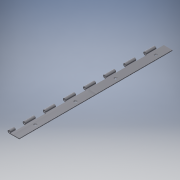
# Autodesk Inventor part: SIDE 1
Saved by Autodesk Inventor 2016 (Build 200138000, 138)
## iProperties
Created: 2015-09-17
Part Number: SIDE 1
Material: Steel, Mild
Document SubType Name: Modeling
Designer: testing
Density: 7.85 g/cm^3
Appearance: Metal-Steel
Mass: 86.1353 g
Surface Area: 160.581 cm^2
Volume: 10.9727 cm^3
Author: testing
Autodesk Inventor part; units mm, degrees
ref_plane "YZ Plane" through (0, 0, 0) normal (1, 0, 0) x (0, 1, 0)
ref_plane "XZ Plane" through (0, 0, 0) normal (0, 1, 0) x (-1, 0, 0)
ref_plane "XY Plane" through (0, 0, 0) normal (0, 0, 1) x (1, 0, 0)
sketch "Sketch2" plane through (0, 0, 0) normal (0, 1, 0) x (-1, 0, 0)
  arc A0 (0, -1.5) -> (-1.3365, -0.681) centre (0, 0) ccw
  arc A1 (0, -3) -> (-2.673, -1.362) centre (0, 0) ccw
  line L0 (0, -3) -> (-20, -3)
  line L1 (-20, -3) -> (-20, -1.5)
  line L2 (-20, -1.5) -> (0, -1.5)
  line L3 (-1.3365, -0.681) -> (-2.673, -1.362)
  dimension "d0" = 1.5
  dimension "d1" = 1.5
  dimension "d2" = 20
  dimension "d3" = 3
  dimension "d4" = 27
  constraints: 8 end point, 4 point on circle, 3 coincident, 2 centre point, 1 horizontal, 1 parallel, 1 perpendicular, 1 point on line, 1 tangent
  measures "d0" distance of L0.end L1.end
  measures "d1" radial gap between concentric circles of A1 A0
  measures "d2" distance from line of point (0, 0) L1
  measures "d3" diameter of A0
  measures "d4" angle of L2 L3
extrude "Extrusion1" add sketch "Sketch2" along normal blind 304.8
sketch "Sketch3" plane through (20, 0, -3) normal (0, 0, -1) x (-1, 0, 0)
  line L0 (0, 0) -> (20, 0) projected
  line L1 (23, 30) -> (17, 30)
  line L2 (17, 30) -> (17, 10)
  line L3 (17, 10) -> (23, 10)
  line L4 (23, 10) -> (23, 30)
  line L5 (17, 0) -> (17, 304.8) projected
  dimension "d7" = 10
  dimension "d8" = 20
  dimension "d9" = 6
  constraints: 8 end point, 2 parallel, 1 horizontal, 1 perpendicular, 1 point on line
  measures "d7" distance between parallel lines of L3 L0
  measures "d8" distance of L3.end L1.start
  measures "d9" distance of L2.end L3.end
extrude "Extrusion2" cut sketch "Sketch3" against normal through all
pattern_linear "Rectangular Pattern1" count 25 spacing 40 along (0, 1, 0) of "Extrusion2"
sketch "Sketch4" plane through (20, 0, -1.5) normal (0, 0, 1) x (1, 0, 0)
  line L0 (-20, 70) -> (-20, 90) projected
  line L1 (-20, 70) -> (-20, 90) projected
  line L2 (-20, 70) -> (-20, 90) projected
  line L3 (-20, 70) -> (-20, 90) projected
  line L4 (-20, 70) -> (-20, 90) projected
  line L5 (-20, 70) -> (-20, 90) projected
  line L6 (-20, 70) -> (-20, 90) projected
  line L7 (-20, 70) -> (-20, 90) projected
  line L8 (-20, 270) -> (-20, 290) projected
  line L9 (-20, 190) -> (-20, 210) projected
  line L10 (-20, 110) -> (-20, 130) projected
  line L11 (-20, 30) -> (-20, 50) projected
  line L12 (0, 0) -> (0, 304.8) projected
  point P0 (-20, 930)
  point P1 (-20, 910)
  point P2 (-20, 850)
  point P3 (-20, 830)
  point P4 (-20, 770)
  point P5 (-20, 750)
  point P6 (-20, 690)
  point P7 (-20, 670)
  point P8 (-20, 610)
  point P9 (-20, 590)
  point P10 (-20, 530)
  point P11 (-20, 510)
  point P12 (-20, 450)
  point P13 (-20, 430)
  point P14 (-20, 370)
  point P15 (-20, 350)
  point P16 (-8, 40)
  point P17 (-8, 120)
  point P18 (-8, 200)
  point P19 (-8, 280)
  point P20 (-8, 360)
  point P21 (-8, 440)
  point P22 (-8, 520)
  point P23 (-8, 600)
  point P24 (-8, 680)
  point P25 (-8, 760)
  point P26 (-8, 840)
  point P27 (-8, 920)
  point P28 (-20, 40)
  point P29 (-20, 120)
  point P30 (-20, 200)
  point P31 (-20, 280)
  point P32 (-20, 360)
  point P33 (-20, 440)
  point P34 (-20, 520)
  point P35 (-20, 600)
  point P36 (-20, 680)
  point P37 (-20, 760)
  point P38 (-20, 840)
  point P39 (-20, 920)
  dimension "d15" = 8
  constraints: 12 horizontal alignment, 11 vertical alignment, 8 point on line, 4 midpoint
  measures "d15" distance from line of L12 point (-8, 40)
hole "Hole1" at (12, 40, -1.5) at (12, 120, -1.5) at (12, 200, -1.5) at (12, 280, -1.5) at (12, 360, -1.5) at (12, 440, -1.5) at (12, 520, -1.5) at (12, 600, -1.5) at (12, 680, -1.5) at (12, 760, -1.5) at (12, 840, -1.5) at (12, 920, -1.5) direction (0, 0, -1) diameter 3 end through all countersink diameter 6 countersink angle 90
equation "\"d1\" = d0"
body "Solid1"
